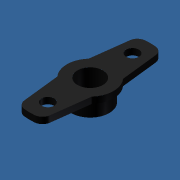
# Autodesk Inventor part: acople para eje falso
Saved by Autodesk Inventor 2014 (Build 180170000, 170)
## iProperties
Created: 2010-09-11
Part Number: acople para eje falso
Document SubType Name: Modeling
Designer: LEFO
Density: 1 g/cm^3
Material: Generic
Appearance: Glossy - Black
Mass: 0.38618 g
Surface Area: 6.72198 cm^2
Volume: 0.38618 cm^3
Author: LEFO
Autodesk Inventor part; units mm, degrees
note: some values were not read from the file. Chosen so that the rebuilt part matches the saved one: sketch regions of "Extrusion1"; sketch regions of "Extrusion2".
ref_plane "YZ Plane" through (0, 0, 0) normal (1, 0, 0) x (0, 1, 0)
ref_plane "XZ Plane" through (0, 0, 0) normal (0, 1, 0) x (-1, 0, 0)
ref_plane "XY Plane" through (0, 0, 0) normal (0, 0, 1) x (1, 0, 0)
sketch "Sketch1" plane through (0, 0, 0) normal (0, 0, 1) x (1, 0, 0)
  circle A0 centre (0, 0.0481) radius 3
  circle A1 centre (0, 0.0481) radius 1.5
  circle A2 centre (0, 0.0481) radius 5.5
  arc A3 (2.6218, 17.0122) -> (-2.3779, 17.0481) centre (0.1221, 17.0481) ccw
  line L0 (0.1221, 17.0481) -> (-2.3779, 17.0481) construction
  line L1 (0.1221, 17.0481) -> (2.6221, 17.0481) construction
  line L2 (2.6221, 17.0481) -> (0.1221, 17.0481) construction
  line L3 (-2.3779, 17.0481) -> (-4.4642, 0.6149)
  line L4 (0.1221, 17.0481) -> (0, 0.0481) construction
  line L5 (2.6218, 17.0122) -> (4.4718, 0.5507)
  line L6 (0, 0.0481) -> (-9.4947, 0.1163) construction
  arc A4 (-2.6218, -16.916) -> (2.3779, -16.9519) centre (-0.1221, -16.9519) ccw
  line L7 (-2.6218, -16.916) -> (-4.4718, -0.4544)
  line L8 (2.3779, -16.9519) -> (4.4642, -0.5186)
  arc A5 (-4.4642, 0.6149) -> (-4.4718, -0.4544) centre (0, 0.0481) ccw
  arc A6 (4.4642, -0.5186) -> (4.4718, 0.5507) centre (0, 0.0481) ccw
  circle A7 centre (0, 0.0481) radius 4.5
  dimension "d1" = 3
  dimension "d2" = 6
  dimension "d4" = 11
  dimension "d5" = 5
  dimension "d6" = 17
  dimension "d8" = 16.5652
  dimension "d9" = 16.5652
  dimension "d10" = 97.235
  dimension "d20" = 13.9277
  constraints: 18 end point, 9 point on circle, 8 centre point, 7 symmetric about line, 4 coincident, 2 collinear, 2 tangent, 1 horizontal, 1 perpendicular, 1 other
  measures "d1" diameter of A1
  measures "d2" diameter of A0
  measures "d4" diameter of A2
  measures "d5" diameter of A3
  measures "d6" vertical distance of L0.start A0.centre
  measures "d8" distance of L0.end L3.end
  measures "d9" distance of L5.start L5.end
  measures "d10" angle of L0 L3
  measures "d20" distance from line of L6.end L5
extrude "Extrusion1" add sketch "Sketch1" along normal blind 1.5 contours L5 A7 L3 A2 | A2 L3 A3 L5 | L8 A4 L7 A2 | A2 L7 A7 L8 | A6 A7 A5
extrude "Extrusion2" add sketch "Sketch1" along normal blind 1.5 contours A2 L8 A6 L5 | L5 A7 L3 A2 | A2 L7 A7 L8 | L3 A5 L7 A2 | A6 A7 A5
extrude "Extrusion3" add sketch "Sketch1" against normal blind 3.5 contours A6 A7 A5
extrude "Extrusion4" add sketch "Sketch1" along normal blind 1.5 contours A0
sketch "Sketch2" plane through (0, 0, 1.5) normal (0, 0, 1) x (1, 0, 0)
  circle A0 centre (0, 0.0481) radius 3 projected
  circle A1 centre (0, 10.0481) radius 1.5
  circle A2 centre (0, -9.9519) radius 1.5
  dimension "d25" = 3
  dimension "d26" = 3
  dimension "d29" = 10
  dimension "d30" = 10
  constraints: 2 centre point, 2 vertical alignment
  measures "d25" diameter of A2
  measures "d26" diameter of A1
  measures "d29" distance of A2.centre A0.centre
  measures "d30" distance of A0.centre A1.centre
extrude "Extrusion5" cut sketch "Sketch2" against normal blind 2 contours A1 | A2
sketch "Sketch3" plane through (0, 0.0481, 0) normal (0, 0, -1) x (-1, 0, 0)
  circle A0 centre (0, 0) radius 1.5 projected
  circle A1 centre (0, 0) radius 3 projected
  point P0 (0, -0.0481)
extrude "Extrusion6" cut sketch "Sketch3" against normal up to next
sketch "Sketch4" plane through (0, 0, 1.5) normal (0, 0, 1) x (1, 0, 0)
  circle A0 centre (0, -9.9519) radius 1.5 projected
  circle A1 centre (0, 10.0481) radius 1.5 projected
  line L0 (2.6218, 17.0122) -> (4.1187, 3.6932) projected
  arc A2 (2.6218, 17.0122) -> (-2.3779, 17.0481) centre (0.1221, 17.0481) ccw projected
  line L1 (-4.0659, 3.752) -> (-2.3779, 17.0481) projected
  line L2 (-2.6218, -16.916) -> (-4.1187, -3.5969) projected
  arc A3 (-2.6218, -16.916) -> (2.3779, -16.9519) centre (-0.1221, -16.9519) ccw projected
  line L3 (4.0659, -3.6557) -> (2.3779, -16.9519) projected
  line L4 (0.1221, 17.0481) -> (0, 10.0481) construction
  line L5 (0, -9.9519) -> (-0.1221, -16.9519) construction
  arc A4 (-2.9596, -13.91) -> (2.7589, -13.9512) centre (0, 0) ccw
  arc A5 (2.9707, 13.9077) -> (-2.7714, 13.9487) centre (0, 0) ccw
  constraints: 4 end point, 4 point on circle, 4 point on line, 2 centre point, 1 coincident, 1 parallel
extrude "Extrusion7" cut sketch "Sketch4" against normal up to next contours L0 A5 L1 A2 | L2 A4 L3 A3
fillet "Fillet1" radius 2 4 edges at (2.7589, -13.9512, 0.75) (-2.9596, -13.91, 0.75) (2.9707, 13.9077, 0.75) (-2.7714, 13.9487, 0.75)
body "Solid1"
